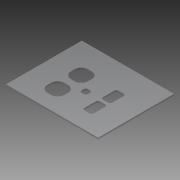
# Autodesk Inventor part: plate_base
Saved by Autodesk Inventor 2014 SP1 (Build 180222100, 222)
## iProperties
Created: 2016-09-05
Part Number: plate_base
Material: PET Plastic
Document SubType Name: Modeling
Designer: tguillod
Density: 1.541 g/cm^3
Appearance: Polycarbonate - Clear
Author: tguillod
Autodesk Inventor part; units mm, degrees
ref_plane "YZ Plane" through (0, 0, 0) normal (1, 0, 0) x (0, 1, 0)
ref_plane "XZ Plane" through (0, 0, 0) normal (0, 1, 0) x (-1, 0, 0)
ref_plane "XY Plane" through (0, 0, 0) normal (0, 0, 1) x (1, 0, 0)
sketch "Sketch1" plane through (0, 0, 0) normal (0, 0, 1) x (1, 0, 0)
  line L0 (0, 0) -> (177.5, 0)
  line L1 (177.5, 0) -> (177.5, 146)
  line L2 (177.5, 146) -> (0, 146)
  line L3 (0, 146) -> (0, 0)
  dimension "d0" = 177.5
  dimension "d1" = 146
  constraints: 8 end point, 2 parallel, 1 horizontal, 1 perpendicular
  measures "d0" distance of L1.end L2.end
  measures "d1" distance of L0.end L1.end
extrude "Extrusion1" add sketch "Sketch1" along normal blind 3
sketch "Sketch4" plane through (0, 0, 3) normal (0, 0, 1) x (1, 0, 0)
  line L0 (0, 0) -> (177.5, 0) projected
  line L1 (177.5, 0) -> (177.5, 146) projected
  line L2 (177.5, 146) -> (0, 146) projected
  line L3 (0, 146) -> (0, 0) projected
  line L4 (40.75, 104.25) -> (73.75, 104.25)
  line L5 (73.75, 104.25) -> (73.75, 71.25)
  line L6 (73.75, 71.25) -> (40.75, 71.25)
  line L7 (40.75, 71.25) -> (40.75, 104.25)
  line L8 (40.75, 58.75) -> (73.75, 58.75)
  line L9 (73.75, 58.75) -> (73.75, 25.75)
  line L10 (73.75, 25.75) -> (40.75, 25.75)
  line L11 (40.75, 25.75) -> (40.75, 58.75)
  line L12 (114.75, 97.75) -> (132.75, 97.75)
  line L13 (132.75, 97.75) -> (132.75, 68)
  line L14 (132.75, 68) -> (114.75, 68)
  line L15 (114.75, 68) -> (114.75, 97.75)
  line L16 (114.75, 62) -> (132.75, 62)
  line L17 (132.75, 62) -> (132.75, 32.25)
  line L18 (132.75, 32.25) -> (114.75, 32.25)
  line L19 (114.75, 32.25) -> (114.75, 62)
  line L20 (82.75, 71) -> (94.75, 71)
  line L21 (94.75, 71) -> (94.75, 59)
  line L22 (94.75, 59) -> (82.75, 59)
  line L23 (82.75, 59) -> (82.75, 71)
  dimension "d37" = 33
  dimension "d38" = 33
  dimension "d39" = 12
  dimension "d40" = 12
  dimension "d41" = 29.75
  dimension "d42" = 18
  dimension "d43" = 40.75
  dimension "d44" = 41.75
  dimension "d45" = 25.75
  dimension "d46" = 82.75
  dimension "d48" = 44.75
  dimension "d49" = 48.25
  dimension "d50" = 32.25
  dimension "d53" = 59
  constraints: 40 end point, 10 parallel, 5 horizontal, 5 perpendicular, 4 equal length, 2 collinear
  measures "d37" distance of L4.start L4.end
  measures "d38" distance of L4.end L5.end
  measures "d39" distance of L20.start L20.end
  measures "d40" distance of L22.end L20.start
  measures "d41" distance of L12.end L13.end
  measures "d42" distance of L12.start L12.end
  measures "d43" distance between parallel lines of L3 L7
  measures "d44" distance between parallel lines of L2 L4
  measures "d45" distance between parallel lines of L0 L10
  measures "d46" distance between parallel lines of L3 L23
  measures "d48" distance between parallel lines of L13 L1
  measures "d49" distance between parallel lines of L2 L12
  measures "d50" distance between parallel lines of L18 L0
  measures "d53" distance between parallel lines of L22 L0
extrude "Extrusion5" cut sketch "Sketch4" against normal blind 10 contours L4 L5 L6 L7 | L8 L9 L10 L11 | L12 L13 L14 L15 | L16 L17 L18 L19 | L20 L21 L22 L23
fillet "Fillet1" radius 4 12 edges at (114.75, 97.75, 1.5) (82.75, 71, 1.5) (94.75, 59, 1.5) (132.75, 32.25, 1.5) (132.75, 68, 1.5) (132.75, 97.75, 1.5) (114.75, 32.25, 1.5) (114.75, 68, 1.5) (82.75, 59, 1.5) (94.75, 71, 1.5) (114.75, 62, 1.5) (132.75, 62, 1.5)
fillet "Fillet2" radius 13 8 edges at (40.75, 58.75, 1.5) (40.75, 104.25, 1.5) (40.75, 71.25, 1.5) (40.75, 25.75, 1.5) (73.75, 71.25, 1.5) (73.75, 25.75, 1.5) (73.75, 104.25, 1.5) (73.75, 58.75, 1.5)
body "Solid1"
